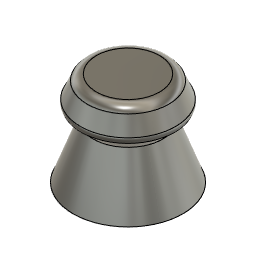
forme1 (Autodesk Fusion 360 design; units mm, degrees)
Autodesk Fusion 360 part; units mm, degrees
sketch "Esquisse2" plane through (0, 0, 0) normal (0, 0, 1) x (1, 0, 0)
  line L0 (-70, 0) -> (-98.2998, 28.2688)
  line L1 (-98.2998, 28.2688) -> (-76.4677, 78.2688)
  line L2 (-76.4677, 78.2688) -> (0, 78.2688)
  line L3 (0, 78.2688) -> (0, 0)
  line L4 (-70, 0) -> (-110, -110)
  line L5 (-110, -110) -> (0, -110)
  line L6 (0, -110) -> (0, 0)
  dimension "d4" = 40
  dimension "d5" = 70
  dimension "d6" = 50
  dimension "d12" = 110
  constraint horizontal L2
  constraint coincident L3.end L6.end
  measures "d4" distance of L0.start L0.end
  measures "d5" distance of L3.end L0.start
  measures "d6" vertical distance of L0.end L1.end
  measures "d12" vertical distance of L0.start L4.end
revolve "Révolution1" add sketch "Esquisse2" angle 360 about axis through (0, 78.2688, 0) along (0, -1, 0)
fillet "Congé1" radius 10 1 edges at (-91.6476, 28.2688, 35.5467)
fillet "Congé2" radius 20 1 edges at (-71.293, 78.2688, 27.6519)
move_body "Déplacer1" bodies 1 to x (1, 0, 0) y (0, 1, 0) z (0, 0, 1) at (0, 110, 0)
